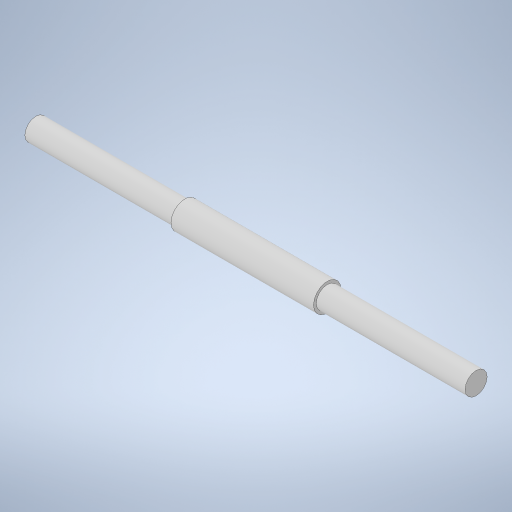
# Autodesk Inventor part: elbow_shaft
Saved by Autodesk Inventor 2024 (Build 280153000, 153)
## iProperties
Created: 2025-08-06
Part Number: elbow_shaft
Material: 一般
Document SubType Name: Modeling
Designer: HosodaLab2
Density: 1 g/cm^3
Appearance: 既定
Author: HosodaLab2
Autodesk Inventor part; units mm, degrees
ref_plane "YZ Plane" through (0, 0, 0) normal (1, 0, 0) x (0, 1, 0)
ref_plane "XZ Plane" through (0, 0, 0) normal (0, 1, 0) x (-1, 0, 0)
ref_plane "XY Plane" through (0, 0, 0) normal (0, 0, 1) x (1, 0, 0)
sketch "スケッチ1" plane through (0, 0, 0) normal (0, 1, 0) x (-1, 0, 0)
  circle A0 centre (0, 0) radius 4
  dimension "d0" = 8
  constraints: 1 centre point, 1 coincident
  measures "d0" diameter of A0
extrude "押し出し1" add sketch "スケッチ1" along normal blind 160
ref_plane "作業平面1" through (0, 80, 0) normal (0, 1, 0) x (1, 0, 0)
sketch "スケッチ2" plane through (0, 80, 0) normal (0, 1, 0) x (1, 0, 0)
  circle A0 centre (0, 0) radius 4 projected
  circle A1 centre (0, 0) radius 5
  dimension "d3" = 10
  constraints: 1 centre point, 1 coincident
  measures "d3" diameter of A1
extrude "押し出し2" add sketch "スケッチ2" along normal blind 25.9 and the other way blind 25.9 contours A0 | A1
sketch "スケッチ3" plane through (0, 80, 0) normal (0, 1, 0) x (1, 0, 0)
  point P0 (0, 0)
